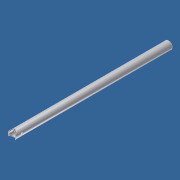
# Autodesk Inventor part: GE-12057-01
Saved by Autodesk Inventor 2012 (Build 160160000, 160)
## iProperties
Created: 2011-08-02
Part Number: GE-12057-01
Document SubType Name: Modeling
Designer: mcyr
Density: 1 g/cm^3
Description: Outer Tube
Material: Default
Title: Outer Tube
Author: mcyr
Autodesk Inventor part; units mm, degrees
ref_plane "YZ Plane" through (0, 0, 0) normal (1, 0, 0) x (0, 1, 0)
ref_plane "XY Plane" through (0, 0, 0) normal (0, 0, 1) x (1, 0, 0)
sketch "Sketch1" plane through (0, 0, 0) normal (0, 0, 1) x (1, 0, 0)
  circle A0 centre (0, 0) radius 17.4625
  circle A1 centre (0, 0) radius 20.6375
  dimension "d0" = 41.275
  dimension "d1" = 34.925
  constraints: 2 centre point, 2 coincident
  measures "d0" diameter of A1
  measures "d1" diameter of A0
extrude "Extrusion1" add sketch "Sketch1" along normal blind 825.5
ref_plane "Work Plane2" through (0, 0, 0) normal (0, 1, 0) x (0, 0, 1)
sketch "Sketch2" plane through (0, 0, 0) normal (0, 1, 0) x (0, 0, 1)
  circle A0 centre (825.4236, 0) radius 16.8275
  point P0 (0, 0)
  dimension "d5" = 33.655
  constraints: 1 centre point
  measures "d5" diameter of A0
extrude "Extrusion2" cut sketch "Sketch2" against normal mid plane 44.45
sketch "Sketch3" plane through (0, 0, 0) normal (1, 0, 0) x (0, 1, 0)
  circle A0 centre (0, 793.75) radius 6.35
  line L0 (-4.6669, 825.5) -> (4.6669, 825.5) projected
  point P0 (0, 0)
  dimension "d8" = 31.75
  dimension "d9" = 12.7
  constraints: 1 centre point
  measures "d8" distance from line of A0.centre L0
  measures "d9" diameter of A0
extrude "Extrusion3" cut sketch "Sketch3" against normal mid plane 44.45
body "Solid1"
